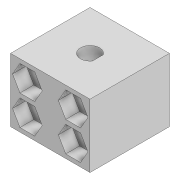
# Autodesk Inventor part: 615456 bevel gear lock A
Saved by Autodesk Inventor 2020 (Build 240168000, 168)
## iProperties
Created: 2019-11-11
Part Number: 615456 bevel gear lock A
Material: Generic
Document SubType Name: Modeling
Designer: ball
Density: 1 g/cm^3
Appearance: Default
Author: ball
Autodesk Inventor part; units mm, degrees
ref_plane "YZ Plane" through (0, 0, 0) normal (1, 0, 0) x (0, 1, 0)
ref_plane "XZ Plane" through (0, 0, 0) normal (0, 1, 0) x (-1, 0, 0)
ref_plane "XY Plane" through (0, 0, 0) normal (0, 0, 1) x (1, 0, 0)
sketch "Sketch1" plane through (0, 0, 0) normal (0, 1, 0) x (-1, 0, 0)
  line L0 (12.5, 12.5) -> (12.5, -12.5)
  line L1 (12.5, -12.5) -> (-12.5, -12.5)
  line L2 (12.5, 12.5) -> (-12.5, 12.5)
  line L3 (-12.5, 12.5) -> (-12.5, -12.5)
  arc A0 (-2.489, -1.6837) -> (-2.489, 1.6837) centre (0, 0) ccw
  line L4 (-2.489, -1.6837) -> (-2.489, 1.6837)
  dimension "d8" = 12.5
  dimension "d9" = 25
  dimension "d10" = 12.5
  dimension "d11" = 25
  dimension "d12" = 6.01
  dimension "d13" = 2.489
  constraints: 10 end point, 2 point on circle, 1 centre point, 1 coincident, 1 vertical
  measures "d8" distance from line of L1 point (0, 0)
  measures "d9" distance between parallel lines of L2 L1
  measures "d10" distance from line of L0 point (0, 0)
  measures "d11" distance between parallel lines of L3 L0
  measures "d12" diameter of A0
  measures "d13" distance from line of L4 point (0, 0)
extrude "Extrusion1" add sketch "Sketch1" along normal blind 20
sketch "Sketch2" plane through (-12.5, 0, 12.5) normal (0, 0, 1) x (1, 0, 0)
  circle A0 centre (5.2959, 14.7041) radius 4.6609 construction
  circle A1 centre (5.2959, 5.2959) radius 4.6609 construction
  circle A2 centre (19.7041, 14.7041) radius 4.6609 construction
  circle A3 centre (19.7041, 5.2959) radius 4.6609 construction
  line L0 (0, 0) -> (0, 20) projected
  line L1 (25, 0) -> (25, 20) projected
  line L2 (0, 20) -> (25, 20) projected
  line L3 (0, 0) -> (25, 0) projected
  line L4 (5.2959, 14.7041) -> (19.7041, 14.7041) construction
  line L5 (5.2959, 5.2959) -> (19.7041, 5.2959) construction
  line L6 (24.365, 14.7041) -> (22.0345, 10.6676)
  line L7 (22.0345, 10.6676) -> (17.3737, 10.6676)
  line L8 (17.3737, 10.6676) -> (15.0432, 14.7041)
  line L9 (15.0432, 14.7041) -> (17.3737, 18.7406)
  line L10 (17.3737, 18.7406) -> (22.0345, 18.7406)
  line L11 (22.0345, 18.7406) -> (24.365, 14.7041)
  line L12 (24.365, 5.2959) -> (22.0345, 1.2594)
  line L13 (22.0345, 1.2594) -> (17.3737, 1.2594)
  line L14 (17.3737, 1.2594) -> (15.0432, 5.2959)
  line L15 (15.0432, 5.2959) -> (17.3737, 9.3324)
  line L16 (17.3737, 9.3324) -> (22.0345, 9.3324)
  line L17 (22.0345, 9.3324) -> (24.365, 5.2959)
  line L18 (9.9568, 5.2959) -> (7.6264, 1.2594)
  line L19 (7.6264, 1.2594) -> (2.9655, 1.2594)
  line L20 (2.9655, 1.2594) -> (0.635, 5.2959)
  line L21 (0.635, 5.2959) -> (2.9654, 9.3324)
  line L22 (2.9654, 9.3324) -> (7.6263, 9.3324)
  line L23 (7.6263, 9.3324) -> (9.9568, 5.2959)
  line L24 (9.9568, 14.7041) -> (7.6264, 10.6676)
  line L25 (7.6264, 10.6676) -> (2.9655, 10.6676)
  line L26 (2.9655, 10.6676) -> (0.635, 14.7041)
  line L27 (0.635, 14.7041) -> (2.9654, 18.7406)
  line L28 (2.9654, 18.7406) -> (7.6263, 18.7406)
  line L29 (7.6263, 18.7406) -> (9.9568, 14.7041)
  point P0 (12.5, 0)
  dimension "d16" = 9.3218
  dimension "d17" = 9.3218
  dimension "d18" = 9.3218
  dimension "d19" = 9.3218
  dimension "d20" = 5.2959
  dimension "d21" = 5.2959
  dimension "d22" = 5.2959
  dimension "d23" = 5.2959
  dimension "d24" = 5.2959
  dimension "d25" = 5.2959
  dimension "d26" = 5.2959
  dimension "d27" = 5.2959
  constraints: 52 end point, 6 coincident, 4 horizontal alignment, 2 point on line, 60 other
  measures "d20" distance from line of L4.start L0
  measures "d21" distance from line of L1 L4.end
  measures "d22" distance from line of L2 L4.start
  measures "d23" distance from line of L2 L4.end
  measures "d24" distance from line of L3 L5.start
  measures "d25" distance from line of L3 L5.end
  measures "d26" distance from line of L0 L5.start
  measures "d27" distance from line of L1 L5.end
sketch "Sketch3" plane through (12.5, 0, -12.5) normal (0, 0, -1) x (-1, 0, 0)
  circle A0 centre (5.2959, 14.7041) radius 1.9304
  line L0 (0, 20) -> (25, 20) projected
  line L1 (0, 0) -> (0, 20) projected
  circle A1 centre (5.2959, 5.2959) radius 1.9304
  line L2 (0, 0) -> (25, 0) projected
  circle A2 centre (19.7041, 14.7041) radius 1.9304
  line L3 (25, 0) -> (25, 20) projected
  circle A3 centre (19.7041, 5.2959) radius 1.9304
  point P0 (12.5, 0)
  dimension "d28" = 3.8608
  dimension "d29" = 5.2959
  dimension "d30" = 5.2959
  dimension "d31" = 3.8608
  dimension "d32" = 5.2959
  dimension "d33" = 5.2959
  dimension "d34" = 3.8608
  dimension "d35" = 5.2959
  dimension "d36" = 5.2959
  dimension "d37" = 3.8608
  dimension "d38" = 5.2959
  dimension "d39" = 5.2959
  constraints: 4 centre point
  measures "d28" diameter of A0
  measures "d29" distance from line of L0 A0.centre
  measures "d30" distance from line of L1 A0.centre
  measures "d31" diameter of A1
  measures "d32" distance from line of L2 A1.centre
  measures "d33" distance from line of L1 A1.centre
  measures "d34" diameter of A2
  measures "d35" distance from line of L3 A2.centre
  measures "d36" distance from line of L0 A2.centre
  measures "d37" diameter of A3
  measures "d38" distance from line of L2 A3.centre
  measures "d39" distance from line of L3 A3.centre
extrude "6-32Holes" cut sketch "Sketch3" against normal through all contours A0 | A1 | A2 | A3
extrude "NutWells" cut sketch "Sketch2" against normal blind 4.3688 contours L6 L7 L8 L9 L10 L11 | L12 L13 L14 L15 L16 L17 | L18 L19 L20 L21 L22 L23 | L24 L25 L26 L27 L28 L29
equation "\"d8\" = 0.5 * d9"
equation "\"d10\" = 0.5 * d11"
equation "\"d20\" = d21"
equation "\"d22\" = d23"
equation "\"d24\" = d23"
equation "\"d25\" = d23"
equation "\"d26\" = d21"
equation "\"d27\" = d21"
equation "\"d29\" = d23"
equation "\"d30\" = d21"
equation "\"d31\" = d28"
equation "\"d32\" = d23"
equation "\"d33\" = d21"
equation "\"d34\" = d28"
equation "\"d35\" = d21"
equation "\"d36\" = d23"
equation "\"d37\" = d28"
equation "\"d38\" = d23"
equation "\"d39\" = d21"
body "Solid1"
